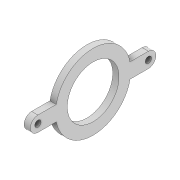
# Autodesk Inventor part: Sujetador_Rodamiento
Saved by Autodesk Inventor 2021 (Build 250183000, 183)
## iProperties
Created: 2022-02-11
Part Number: Sujetador_Rodamiento
Material: Generic
Document SubType Name: Modeling
Designer: Santiago
Density: 1 g/cm^3
Appearance: Default
Author: Santiago
Autodesk Inventor part; units mm, degrees
ref_plane "YZ Plane" through (0, 0, 0) normal (1, 0, 0) x (0, 1, 0)
ref_plane "XZ Plane" through (0, 0, 0) normal (0, 1, 0) x (-1, 0, 0)
ref_plane "XY Plane" through (0, 0, 0) normal (0, 0, 1) x (1, 0, 0)
sketch "Sketch1" plane through (0, 0, 0) normal (1, 0, 0) x (0, 1, 0)
  circle A0 centre (0, 0) radius 10
  circle A1 centre (0, 0) radius 20.6375
  line L0 (0, 0) -> (0, 44)
  circle A2 centre (0, 44) radius 2.5
  line L1 (20.6375, 0) -> (-20.6375, 0)
  arc A3 (6, 44) -> (-6, 44) centre (0, 44) ccw
  line L2 (6, 44) -> (6, 29.3939)
  line L3 (-6, 44) -> (-6, 29.3939)
  circle A4 centre (0, -44) radius 2.5
  arc A5 (-6, -44) -> (6, -44) centre (0, -44) ccw
  line L4 (6, -44) -> (6, -29.3939)
  line L5 (-6, -44) -> (-6, -29.3939)
  arc A6 (-6, 29.3939) -> (-6, -29.3939) centre (0, 0) ccw
  arc A7 (6, -29.3939) -> (6, 29.3939) centre (0, 0) ccw
  dimension "d0" = 20
  dimension "d1" = 41.275
  dimension "d5" = 44
  dimension "d6" = 5
  dimension "d7" = 12
  constraints: 12 end point, 10 point on circle, 8 centre point, 6 coincident, 6 symmetric about line, 2 vertical, 1 horizontal, 1 parallel, 1 tangent, 2 other
  measures "d0" diameter of A0
  measures "d1" diameter of A1
  measures "d5" distance of L0.start L0.end
  measures "d6" diameter of A2
  measures "d7" diameter of A3
extrude "Extrusion1" add sketch "Sketch1" along normal blind 5
body "Solid1"
